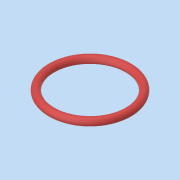
# Autodesk Inventor part: ORingA50_1.296ID_1.574OD
Saved by Autodesk Inventor 2017 (Build 210142000, 142)
## iProperties
Created: 2016-10-16
Part Number: ORingA50_1.296ID_1.574OD
Material: Rubber, Silicone
Document SubType Name: Modeling
Designer: techn
Density: 1.25 g/cm^3
Appearance: Smooth - Red
Author: techn
Autodesk Inventor part; units mm, degrees
ref_plane "YZ Plane" through (0, 0, 0) normal (1, 0, 0) x (0, 1, 0)
ref_plane "XZ Plane" through (0, 0, 0) normal (0, 1, 0) x (-1, 0, 0)
ref_plane "XY Plane" through (0, 0, 0) normal (0, 0, 1) x (1, 0, 0)
sketch "Sketch1" plane through (0, 0, 0) normal (0, 0, 1) x (1, 0, 0)
  circle A0 centre (18.2245, 0) radius 1.7653
  line L0 (0, 0) -> (0, 8.4357)
  dimension "d0" = 3.5306
  dimension "d1" = 18.2245
  constraints: 2 end point, 1 centre point, 1 vertical
  measures "d0" diameter of A0
  measures "d1" distance from line of A0.centre L0
revolve "Revolution1" add sketch "Sketch1" angle 360 about axis through (0, 0, 0) along (0, 1, 0)
body "Solid1"
